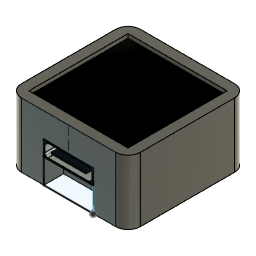
M5_ATOM_MATRIX_ESP32 v2 (Autodesk Fusion 360 design; units mm, degrees)
Autodesk Fusion 360 part; units mm, degrees
sketch "Esquisse1" plane through (0, 0, 0) normal (0, 0, 1) x (1, 0, 0)
  line L0 (0, 50) -> (24, 50)
  line L1 (24, 50) -> (24, 74)
  line L2 (24, 74) -> (0, 74)
  line L3 (0, 74) -> (0, 50)
  dimension "d1" = 24
  dimension "d2" = 24
  constraint horizontal L0
  constraint vertical L1
  constraint horizontal L2
  constraint vertical L3
  measures "d1" distance of L0.start L0.end
  measures "d2" distance of L0.start L2.end
extrude "Extrusion1" add sketch "Esquisse1" along normal blind 13 makes body 1
fillet "Congé1" radius 2.5 4 edges at (0, 50, 6.5) (24, 50, 6.5) (0, 74, 6.5) (24, 74, 6.5) on bodies 1
sketch "Esquisse2" plane through (0, 0, 13) normal (0, 0, 1) x (-1, 0, 0)
  arc A0 (-24, -71.5) -> (-21.5, -74) centre (-21.5, -71.5) ccw
  line L0 (-21.5, -74) -> (-2.5, -74)
  arc A1 (-2.5, -74) -> (0, -71.5) centre (-2.5, -71.5) ccw
  line L1 (0, -71.5) -> (0, -52.5)
  arc A2 (0, -52.5) -> (-2.5, -50) centre (-2.5, -52.5) ccw
  line L2 (-2.5, -50) -> (-21.5, -50)
  arc A3 (-21.5, -50) -> (-24, -52.5) centre (-21.5, -52.5) ccw
  line L3 (-24, -52.5) -> (-24, -71.5)
  line L4 (-2, -72) -> (-22, -72)
  line L5 (-22, -72) -> (-22, -52)
  line L6 (-22, -52) -> (-2, -52)
  line L7 (-2, -52) -> (-2, -72)
  constraint horizontal L4
  constraint vertical L5
  constraint horizontal L6
  constraint vertical L7
extrude "Extrusion2" cut sketch "Esquisse2" against normal blind 1 contours L4 L5 L6 L7 bodies 1
sketch "Esquisse4" plane through (0, 50, 0) normal (0, -1, 0) x (1, 0, 0)
  line L0 (21.5, 0) -> (21.5, 13)
  line L1 (21.5, 13) -> (2.5, 13)
  line L2 (2.5, 13) -> (2.5, 0)
  line L3 (2.5, 0) -> (21.5, 0)
  line L4 (12, 13) -> (12, 8) construction
  line L5 (7, 8) -> (17, 8)
  line L6 (17, 8) -> (17, 5)
  line L7 (17, 5) -> (7, 5)
  line L8 (7, 5) -> (7, 8)
  line L9 (7, 5) -> (17, 5)
  line L10 (17, 5) -> (17, 0)
  line L11 (17, 0) -> (7, 0)
  line L12 (7, 0) -> (7, 5)
  dimension "d9" = 5
  dimension "d10" = 10
  dimension "d11" = 3
  constraint midpoint L1 L4.start
  constraint perpendicular L1 L4
  constraint horizontal L5
  constraint vertical L6
  constraint horizontal L7
  constraint vertical L8
  constraint midpoint L4.end L5
  constraint horizontal L9
  constraint vertical L10
  constraint horizontal L11
  constraint vertical L12
  constraint coincident L3 L10.end
  measures "d9" distance of L4.start L4.end
  measures "d10" distance of L5.start L5.end
  measures "d11" distance of L5.start L7.end
extrude "Extrusion3" cut sketch "Esquisse4" against normal blind 4 contours L5 L6 L7 L8 L9 bodies 1
extrude "Extrusion4" cut sketch "Esquisse4" against normal blind 4 contours L3 L7 L9 L10 L11 L12 bodies 1
sketch "Esquisse5" plane through (0, 50, 0) normal (0, -1, 0) x (1, 0, 0)
  line L0 (7.8136, 7.8653) -> (16.1255, 7.8653)
  line L1 (16.8255, 7.1653) -> (16.8255, 5.8)
  line L2 (16.1255, 5.1) -> (7.8046, 5.1)
  line L3 (7.1046, 5.8046) -> (7.1136, 7.1699)
  line L4 (8.5, 6.5) -> (15.5, 6.5)
  line L5 (15.5, 6.5) -> (15.5, 6.2135)
  line L6 (15.5, 6.2135) -> (8.5, 6.2135)
  line L7 (8.5, 6.2135) -> (8.5, 6.5)
  arc A0 (7.8136, 7.8653) -> (7.1136, 7.1699) centre (7.8136, 7.1653) ccw
  arc A1 (7.1046, 5.8046) -> (7.8046, 5.1) centre (7.8046, 5.8) ccw
  arc A2 (16.8255, 7.1653) -> (16.1255, 7.8653) centre (16.1255, 7.1653) ccw
  arc A3 (16.1255, 5.1) -> (16.8255, 5.8) centre (16.1255, 5.8) ccw
  dimension "d18" = 0.7
  constraint horizontal L0
  constraint perpendicular L0 L1
  constraint perpendicular L1 L2
  constraint horizontal L4
  constraint vertical L5
  constraint horizontal L6
  constraint vertical L7
  constraint tangent L3 A0
  constraint tangent L0 A0
  constraint tangent L2 A1
  constraint tangent L3 A1
  constraint equal A0 A1
  constraint tangent L0 A2
  constraint tangent L1 A2
  constraint equal A0 A2
  constraint tangent L1 A3
  constraint tangent L2 A3
  constraint equal A0 A3
  measures "d18" radius of A0
extrude "Extrusion7" add sketch "Esquisse5" against normal blind 4 separate body contours L0 L1 L2 L3 A0 A1 A2 A3 | L4 L5 L6 L7 makes body 2
shell "Coque2" thickness 0.1 removed faces 1 at (10.5812, 50, 6.0218) on bodies 2
extrude "Extrusion8" add sketch "Esquisse5" against normal blind 4 separate body contours L4 L5 L6 L7 makes body 3
sketch "Esquisse6" plane through (0, 0, 0) normal (0, 0, -1) x (1, 0, 0)
  line L0 (17, -50) -> (17, -54)
  line L1 (17, -54) -> (7, -54)
  line L2 (7, -54) -> (7, -50)
  line L3 (7, -50) -> (2.5, -50)
  arc A0 (2.5, -50) -> (0, -52.5) centre (2.5, -52.5) ccw
  line L4 (0, -52.5) -> (0, -71.5)
  arc A1 (0, -71.5) -> (2.5, -74) centre (2.5, -71.5) ccw
  line L5 (2.5, -74) -> (21.5, -74)
  arc A2 (21.5, -74) -> (24, -71.5) centre (21.5, -71.5) ccw
  line L6 (24, -71.5) -> (24, -52.5)
  arc A3 (24, -52.5) -> (21.5, -50) centre (21.5, -52.5) ccw
  line L7 (21.5, -50) -> (17, -50)
  line L8 (0, -53) -> (3, -53)
  line L9 (3.0754, -50) -> (3.0754, -53)
  line L10 (3.0754, -53) -> (5.5754, -53)
  line L11 (5.5754, -53) -> (5.5754, -63.16)
  line L12 (5.5754, -63.16) -> (3.0754, -63.16)
  line L13 (3.0754, -63.16) -> (3.0754, -53)
  line L14 (24, -53) -> (21, -53)
  line L15 (21, -53) -> (18.5, -53)
  line L16 (18.5, -53) -> (18.5, -65.7)
  line L17 (18.5, -65.7) -> (21, -65.7)
  line L18 (21, -65.7) -> (21, -53)
  dimension "d27" = 3
  dimension "d28" = 3
  dimension "d29" = 2.5
  dimension "d30" = 10.16
  dimension "d31" = 3
  dimension "d32" = 2.5
  dimension "d33" = 12.7
  constraint coincident L4 L8.start
  constraint perpendicular L4 L8
  constraint coincident L3 L9.start
  constraint perpendicular L8 L9
  constraint horizontal L10
  constraint vertical L11
  constraint horizontal L12
  constraint vertical L13
  constraint coincident L6 L14.start
  constraint perpendicular L6 L14
  constraint horizontal L15
  constraint vertical L16
  constraint horizontal L17
  constraint vertical L18
  measures "d27" distance of L8.start L8.end
  measures "d28" distance of L9.start L9.end
  measures "d29" distance of L9.end L10.end
  measures "d30" distance of L9.end L12.end
  measures "d31" distance of L14.start L14.end
  measures "d32" distance of L14.end L15.end
  measures "d33" distance of L14.end L17.end
extrude "Extrusion9" cut sketch "Esquisse6" against normal blind 8.5 contours L10 L11 L12 L13 | L15 L16 L17 L18 bodies 1
extrude "Extrusion10" add 1 faces at (8.6667, 65.3333, 12) along direction (0, 0, 1) blind 0.2 separate body on bodies 1 makes body 4
equation "d30 = ( 2.54 * 4 ) * 1 mm"
equation "d33 = ( 2.54 * 5 ) * 1 mm"
named bodies: "USB-C", "USB-C_INTERNAL"
